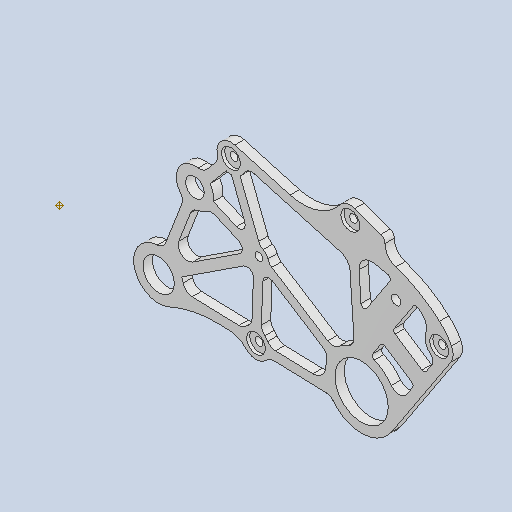
# Autodesk Inventor part: ギア抑え
Saved by Autodesk Inventor 2023 (Build 270158000, 158)
## iProperties
Created: 2022-01-29
Part Number: ギア抑え
Material: Aluminum 2014-T6
Document SubType Name: Modeling
Designer: acps
Density: 2.78927 g/cm^3
Appearance: Satin
Author: acps
Autodesk Inventor part; units mm, degrees
ref_plane "YZ Plane" through (0, 0, 0) normal (1, 0, 0) x (0, 1, 0)
ref_plane "XZ Plane" through (0, 0, 0) normal (0, 1, 0) x (-1, 0, 0)
ref_plane "XY Plane" through (0, 0, 0) normal (0, 0, 1) x (1, 0, 0)
sketch "Sketch4" plane through (0, 0, 0) normal (0, 0, 1) x (1, 0, 0)
  circle A0 centre (58.1571, 43.8132) radius 1.25
  circle A1 centre (46.616, 30) radius 3
  circle A2 centre (35, 0) radius 5.025
  circle A3 centre (67.0906, 21) radius 1.25
  circle A4 centre (67.0906, 21) radius 3
  circle A5 centre (66.1789, -3.483) radius 1.25
  circle A6 centre (58.1571, 43.8132) radius 4.5
  circle A7 centre (66.1789, -3.483) radius 4.5
  circle A8 centre (46.616, 30) radius 6
  circle A9 centre (100, 0) radius 8.525
  circle A10 centre (124.8574, 25) radius 1.25
  circle A11 centre (124.8574, 25) radius 4.5
  circle A12 centre (100, 0) radius 11.525
  circle A13 centre (35, 0) radius 8.025
  line L0 (59.3787, 48.1442) -> (77.1194, 43.1404)
  line L1 (128.6167, 22.5266) -> (109.628, -6.3346)
  line L2 (122.5484, 18.7615) -> (114.5052, 6.5365)
  line L3 (100.7071, 11.5033) -> (100.7003, 11.6011) construction
  line L4 (97.7142, 11.2961) -> (97.7075, 11.3939) construction
  line L5 (68.4738, 18.3379) -> (68.492, 18.3263) construction
  line L6 (70.0876, 20.8669) -> (71.243, 20.1297) construction
  line L7 (67.0906, 21) -> (100, 0) construction
  line L8 (67.0906, 21) -> (124.8574, 25) construction
  line L9 (105.9328, 11.9634) -> (90.1084, 10.8677) construction
  line L10 (100, 0) -> (97.2271, 40.0448) construction
  line L11 (65.705, -7.958) -> (65.6864, -7.956) construction
  line L12 (65.6964, -7.9837) -> (66.1849, -7.983) construction
  line L13 (65.4949, 18.4595) -> (65.4836, 18.1558) construction
  line L14 (67.8357, 0.7009) -> (67.9011, 2.457) construction
  line L15 (67.0906, 21) -> (66.1789, -3.483) construction
  arc A14 (71.4365, 16.4474) -> (68.3621, 14.8358) centre (70.3607, 14.7614) ccw
  line L16 (68.492, 18.3263) -> (68.4928, 18.3479) construction
  line L17 (68.492, 18.3263) -> (71.4365, 16.4474) construction
  line L18 (35, 0) -> (46.616, 30) construction
  line L19 (43.1196, 25.1241) -> (42.4029, 23.2732) construction
  line L20 (39.2454, 6.8101) -> (41.4547, 12.5158) construction
  line L21 (46.616, 30) -> (67.0906, 21) construction
  line L22 (51.3308, 26.289) -> (53.1477, 25.4903) construction
  line L23 (52.538, 29.0354) -> (59.937, 25.783)
  line L24 (61.1008, 40.4096) -> (67.0402, 25.2423)
  line L25 (67.0906, 21) -> (58.1571, 43.8132) construction
  line L26 (58.3073, 39.3157) -> (62.6041, 28.3432)
  arc A15 (59.937, 25.783) -> (62.6041, 28.3432) centre (60.7418, 27.6139) ccw
  line L27 (62.6041, 28.3432) -> (64.7465, 22.8723) construction
  line L28 (59.937, 25.783) -> (65.3157, 23.4187) construction
  line L29 (71.4365, 16.4474) -> (87.5511, 6.1645)
  line L30 (68.3621, 14.8358) -> (68.492, 18.3263) construction
  line L31 (46.616, 30) -> (58.1571, 43.8132) construction
  line L32 (51.492, 33.4964) -> (56.5879, 39.5957)
  line L33 (49.1898, 35.4199) -> (50.4624, 36.943) construction
  arc A16 (58.9156, 37.7626) -> (55.5184, 38.3156) centre (57.0532, 37.0333) ccw
  line L34 (35, 0) -> (67.0906, 21) construction
  line L35 (40.7753, 5.572) -> (45.895, 8.9223) construction
  line L36 (65.738, 18.3222) -> (62.2459, 16.037) construction
  arc A17 (60.8674, 18.7202) -> (60.577, 22.2246) centre (59.7722, 20.3937) ccw
  line L37 (60.577, 22.2246) -> (64.1085, 20.6723) construction
  line L38 (60.8674, 18.7202) -> (64.0952, 20.8325) construction
  arc A18 (65.3396, 14.2891) -> (62.2459, 16.037) centre (63.341, 14.3635) ccw
  line L39 (62.2459, 16.037) -> (42.418, 3.0617)
  line L40 (65.3396, 14.2891) -> (64.9032, 2.5686)
  line L41 (65.4836, 18.1558) -> (65.3396, 14.2891) construction
  circle A19 centre (58.1571, 43.8132) radius 3.025
  circle A20 centre (124.8574, 25) radius 3.025
  circle A21 centre (66.1789, -3.483) radius 3.025
  line L42 (42.994, -0.7047) -> (45.7073, -0.79) construction
  line L43 (70.5412, -2.3784) -> (72.4006, -2.4369) construction
  line L44 (62.6476, 44.1052) -> (65.6368, 43.262) construction
  arc A22 (118.6753, 31.9015) -> (102.5834, 37.8093) centre (98.9344, 3) ccw
  arc A23 (120.5723, 26.3742) -> (118.6753, 31.9015) centre (115.9192, 27.8664) ccw
  arc A24 (103.7268, 37.6704) -> (99.1887, 33.4317) centre (103.1791, 33.708) ccw
  arc A25 (77.1194, 43.1404) -> (93.0418, 48.3811) centre (81.1913, 57.5771) ccw
  circle A26 centre (96.3994, 45.7756) radius 1.25
  circle A27 centre (96.3994, 45.7756) radius 4.25
  arc A28 (122.5484, 18.7615) -> (122.1022, 21.4421) centre (120.8776, 19.8608) ccw
  arc A29 (109.5207, 6.4948) -> (114.5052, 6.5365) centre (111.999, 8.1854) ccw
  line L45 (114.5052, 6.5365) -> (111.3846, 1.7934) construction
  arc A30 (84.3946, -2.8136) -> (88.5086, 0.8792) centre (84.5202, 1.1844) ccw
  line L46 (84.3946, -2.8136) -> (88.86, -2.9539) construction
  arc A31 (107.4852, 44.8614) -> (110.9454, 40.1044) centre (112.4852, 44.8614) ccw
  arc A32 (124.964, 32.0424) -> (110.9454, 40.1044) centre (98.9344, 3) ccw
  arc A33 (128.8264, 27.1206) -> (124.964, 32.0424) centre (112.9503, 18.6382) ccw
  line L47 (97.8537, 49.769) -> (106.1696, 46.7406)
  arc A34 (107.4852, 44.8614) -> (106.1696, 46.7406) centre (105.4852, 44.8614) ccw
  arc A35 (41.4547, 12.5158) -> (45.895, 8.9223) centre (44.2523, 11.4326) ccw
  line L48 (41.4547, 12.5158) -> (45.2005, 22.19)
  line L49 (45.895, 8.9223) -> (60.8674, 18.7202)
  arc A36 (42.8623, 1.6076) -> (45.7073, -0.79) centre (45.8015, 2.2085) ccw
  line L50 (45.7073, -0.79) -> (60.6999, -1.261)
  arc A37 (34.5908, 8.0146) -> (37.2354, 9.9274) centre (34.4378, 11.0107) ccw
  line L51 (37.2354, 9.9274) -> (36.4478, 7.8933) construction
  arc A38 (42.4029, 23.2732) -> (41.9422, 26.2376) centre (39.6053, 24.3565) ccw
  line L52 (42.4029, 23.2732) -> (37.2354, 9.9274)
  arc A39 (47.6454, 35.911) -> (50.4624, 36.943) centre (48.1601, 38.8666) ccw
  line L53 (50.4624, 36.943) -> (53.159, 40.1706)
  arc A40 (65.6368, 43.262) -> (62.1563, 41.7501) centre (64.8224, 40.3747) ccw
  line L54 (65.6368, 43.262) -> (93.3856, 35.4353)
  arc A41 (60.6999, -1.261) -> (62.948, -0.3507) centre (60.7941, 1.7376) ccw
  line L55 (60.6999, -1.261) -> (62.2387, -1.3093) construction
  arc A42 (69.9684, -1.0562) -> (72.4006, -2.4369) centre (72.4948, 0.5617) ccw
  line L56 (72.4006, -2.4369) -> (84.3946, -2.8136)
  arc A43 (63.6147, 0.2149) -> (64.9032, 2.5686) centre (61.9053, 2.6803) ccw
  arc A44 (67.9011, 2.457) -> (69.011, 0.014) centre (70.899, 2.3454) ccw
  line L57 (64.9032, 2.5686) -> (64.8378, 0.8125) construction
  line L58 (67.9011, 2.457) -> (68.3621, 14.8358)
  arc A45 (67.0402, 25.2423) -> (68.4621, 23.6681) centre (69.8336, 26.3362) ccw
  arc A46 (69.9736, 21.8293) -> (71.243, 20.1297) centre (72.8567, 22.6586) ccw
  line L59 (67.0402, 25.2423) -> (67.5399, 23.9662) construction
  line L60 (71.243, 20.1297) -> (89.1649, 8.6934)
  arc A47 (53.159, 40.1706) -> (53.7769, 42.7817) centre (50.8568, 42.0941) ccw
  line L61 (53.159, 40.1706) -> (54.2857, 41.5192) construction
  arc A48 (47.5374, 24.0712) -> (45.2005, 22.19) centre (47.9981, 21.1068) ccw
  arc A49 (53.1477, 25.4903) -> (50.1657, 25.1626) centre (51.9405, 22.744) ccw
  line L62 (45.2005, 22.19) -> (45.9172, 24.0408) construction
  line L63 (53.1477, 25.4903) -> (60.577, 22.2246)
  arc A50 (96.2902, 31.8619) -> (93.3856, 35.4353) centre (92.2997, 31.5855) ccw
  arc A51 (88.8418, 2.8846) -> (87.5511, 6.1645) centre (85.9373, 3.6355) ccw
  arc A52 (89.1649, 8.6934) -> (92.6832, 8.9045) centre (90.7787, 11.2224) ccw
  arc A53 (95.681, 10.6851) -> (97.5496, 13.6737) centre (94.5568, 13.4665) ccw
  arc A54 (100.5424, 13.881) -> (102.8051, 11.1784) centre (103.5353, 14.0882) ccw
  line L64 (87.5511, 6.1645) -> (89.5603, 4.8824) construction
  line L65 (89.1649, 8.6934) -> (91.174, 7.4113) construction
  line L66 (97.7075, 11.3939) -> (97.5496, 13.6737) construction
  line L67 (97.5496, 13.6737) -> (96.2902, 31.8619)
  line L68 (100.7003, 11.6011) -> (100.5424, 13.881) construction
  line L69 (100.5424, 13.881) -> (99.1887, 33.4317)
  circle A55 centre (111.0805, 30.9772) radius 1.5
  arc A56 (109.045, 35.1608) -> (108.4824, 36.6725) centre (108.2096, 35.7104) ccw
  arc A57 (117.9732, 32.3688) -> (116.5938, 32.0793) centre (117.4292, 31.5297) ccw
  line L70 (109.045, 35.1608) -> (101.6472, 23.9169)
  line L71 (116.5938, 32.0793) -> (103.5648, 12.2763)
  arc A58 (103.5648, 12.2763) -> (104.0488, 10.7904) centre (104.4002, 11.7266) ccw
  arc A59 (99.8142, 24.3974) -> (101.6472, 23.9169) centre (100.8118, 24.4665) ccw
  arc A60 (107.4624, 16.381) -> (106.0773, 16.0952) centre (106.9127, 15.5456) ccw
  line L72 (107.4624, 16.381) -> (116.0624, 10.7227)
  arc A61 (116.3482, 9.3377) -> (116.0624, 10.7227) centre (115.5128, 9.8873) ccw
  line L73 (111.877, 28.1536) -> (124.7416, 19.6896) construction
  line L74 (107.3053, 20.0754) -> (119.422, 12.1035) construction
  line L75 (110.7602, 21.3934) -> (119.3603, 15.7351)
  arc A62 (110.4744, 22.7784) -> (110.7602, 21.3934) centre (111.3098, 22.2288) ccw
  arc A63 (119.3603, 15.7351) -> (120.7453, 16.0209) centre (119.9099, 16.5705) ccw
  line L76 (102.8536, 11.9183) -> (111.9722, 5.9189) construction
  circle A64 centre (96.3994, 45.7756) radius 3.025
  arc A65 (56.821, -6.4645) -> (37.4687, -8.6808) centre (53.881, -66.3925) ccw construction
  arc A66 (56.821, -6.4645) -> (59.8142, -6.4542) centre (58.2196, 22.0427) ccw construction
  arc A67 (71.3782, -23.4684) -> (59.8142, -6.4542) centre (60.4847, -18.4355) ccw construction
  arc A68 (54.4173, -4.0651) -> (38.3334, -7.2999) centre (53.2869, -40.0473) ccw
  line L77 (54.4173, -4.0651) -> (57.8446, -4.1727)
  arc A69 (62.8316, -6.4907) -> (57.8446, -4.1727) centre (57.6249, -11.1693) ccw
  arc A70 (71.9175, -5.4232) -> (69.5655, -6.4462) centre (71.8233, -8.4217) ccw
  line L78 (71.9175, -5.4232) -> (88.6522, -5.9489)
  arc A71 (90.9212, -7.0994) -> (88.6522, -5.9489) centre (88.558, -8.9474) ccw
  point P0 (0, 0)
  point P1 (62.6167, 23.75)
  point P2 (63.8469, 21.7439)
  point P3 (63.7276, 4.995)
  point P4 (48.9428, 29.7841)
  point P5 (49.819, 30.1472)
  point P6 (62.9071, 26.3997)
  point P7 (50.9368, 32.3834)
  point P8 (50.8115, 33.0283)
  point P9 (57.8297, 40.9724)
  point P10 (62.9138, 26.4056)
  point P11 (67.612, 23.8643)
  point P12 (65.579, 26.356)
  point P13 (60.2796, 41.5397)
  point P14 (109.8309, 27.4562)
  point P15 (109.8687, 27.322)
  point P16 (93.5994, 9.6725)
  point P17 (91.8321, 9.416)
  point P18 (89.3299, 7.9976)
  point P19 (66.2271, 4.9132)
  point P20 (66.3467, 21.7081)
  point P21 (48.9379, 34.6835)
  point P22 (46.5685, 30.5773)
  point P23 (64.7751, 2.2487)
  point P24 (65.1323, 2.2448)
  point P25 (91.0705, 5.7078)
  point P26 (95.4376, 7.978)
  point P27 (111.7069, 25.6275)
  point P28 (110.5144, 29.861)
  point P29 (60.7307, 44.0105)
  point P30 (55.9361, 42.605)
  point P31 (92.4107, 6.1598)
  point P32 (92.438, 8.4126)
  point P33 (93.6914, 8.3068)
  point P34 (64.5533, 22.7819)
  point P35 (64.4718, 22.8265)
  point P36 (65.6711, 25.0181)
  point P37 (47.5045, 33.0609)
  point P38 (49.0002, 33.3514)
  point P39 (49.5268, 31.5741)
  point P40 (62.6167, 23.75)
  point P41 (63.8469, 21.7439)
  point P42 (63.7276, 4.995)
  point P43 (48.9428, 29.7841)
  point P44 (49.819, 30.1472)
  point P45 (62.9071, 26.3997)
  point P46 (50.9368, 32.3834)
  point P47 (50.8115, 33.0283)
  point P48 (57.8297, 40.9724)
  point P49 (62.9138, 26.4056)
  point P50 (67.612, 23.8643)
  point P51 (65.579, 26.356)
  point P52 (60.2796, 41.5397)
  point P53 (109.8309, 27.4562)
  point P54 (109.8687, 27.322)
  point P55 (93.5994, 9.6725)
  point P56 (91.8321, 9.416)
  point P57 (89.3299, 7.9976)
  point P58 (66.2271, 4.9132)
  point P59 (66.3467, 21.7081)
  point P60 (48.9379, 34.6835)
  point P61 (46.5685, 30.5773)
  point P62 (64.7751, 2.2487)
  point P63 (65.1323, 2.2448)
  point P64 (91.0705, 5.7078)
  point P65 (95.4376, 7.978)
  point P66 (111.7069, 25.6275)
  point P67 (110.5144, 29.861)
  point P68 (60.7307, 44.0105)
  point P69 (55.9361, 42.605)
  point P70 (92.4107, 6.1598)
  point P71 (92.438, 8.4126)
  point P72 (93.6914, 8.3068)
  point P73 (64.5533, 22.7819)
  point P74 (64.4718, 22.8265)
  point P75 (65.6711, 25.0181)
  point P76 (47.5045, 33.0609)
  point P77 (49.0002, 33.3514)
  point P78 (49.5268, 31.5741)
  point P79 (62.6167, 23.75)
  point P80 (63.8469, 21.7439)
  point P81 (63.7276, 4.995)
  point P82 (48.9428, 29.7841)
  point P83 (49.819, 30.1472)
  point P84 (62.9071, 26.3997)
  point P85 (50.9368, 32.3834)
  point P86 (50.8115, 33.0283)
  point P87 (57.8297, 40.9724)
  point P88 (62.9138, 26.4056)
  point P89 (67.612, 23.8643)
  point P90 (65.579, 26.356)
  point P91 (60.2796, 41.5397)
  point P92 (109.8309, 27.4562)
  point P93 (109.8687, 27.322)
  point P94 (93.5994, 9.6725)
  point P95 (91.8321, 9.416)
  point P96 (89.3299, 7.9976)
  point P97 (66.2271, 4.9132)
  point P98 (66.3467, 21.7081)
  point P99 (48.9379, 34.6835)
  point P100 (46.5685, 30.5773)
  point P101 (64.7751, 2.2487)
  point P102 (65.1323, 2.2448)
  point P103 (91.0705, 5.7078)
  point P104 (95.4376, 7.978)
  point P105 (111.7069, 25.6275)
  point P106 (110.5144, 29.861)
  point P107 (60.7307, 44.0105)
  point P108 (55.9361, 42.605)
  point P109 (92.4107, 6.1598)
  point P110 (92.438, 8.4126)
  point P111 (93.6914, 8.3068)
  point P112 (64.5533, 22.7819)
  point P113 (64.4718, 22.8265)
  point P114 (65.6711, 25.0181)
  point P115 (47.5045, 33.0609)
  point P116 (49.0002, 33.3514)
  point P117 (49.5268, 31.5741)
  point P118 (62.6167, 23.75)
  point P119 (63.8469, 21.7439)
  point P120 (63.7276, 4.995)
  point P121 (48.9428, 29.7841)
  point P122 (49.819, 30.1472)
  point P123 (62.9071, 26.3997)
  point P124 (50.9368, 32.3834)
  point P125 (50.8115, 33.0283)
  point P126 (57.8297, 40.9724)
  point P127 (62.9138, 26.4056)
  point P128 (67.612, 23.8643)
  point P129 (65.579, 26.356)
  point P130 (60.2796, 41.5397)
  point P131 (109.8309, 27.4562)
  point P132 (109.8687, 27.322)
  point P133 (93.5994, 9.6725)
  point P134 (91.8321, 9.416)
  point P135 (89.3299, 7.9976)
  point P136 (66.2271, 4.9132)
  point P137 (66.3467, 21.7081)
  point P138 (48.9379, 34.6835)
  point P139 (46.5685, 30.5773)
  point P140 (64.7751, 2.2487)
  point P141 (65.1323, 2.2448)
  point P142 (91.0705, 5.7078)
  point P143 (95.4376, 7.978)
  point P144 (111.7069, 25.6275)
  point P145 (110.5144, 29.861)
  point P146 (60.7307, 44.0105)
  point P147 (55.9361, 42.605)
  point P148 (92.4107, 6.1598)
  point P149 (92.438, 8.4126)
  point P150 (93.6914, 8.3068)
  point P151 (64.5533, 22.7819)
  point P152 (64.4718, 22.8265)
  point P153 (65.6711, 25.0181)
  point P154 (47.5045, 33.0609)
  point P155 (49.0002, 33.3514)
  point P156 (49.5268, 31.5741)
  point P157 (62.6167, 23.75)
  point P158 (63.8469, 21.7439)
  point P159 (63.7276, 4.995)
  point P160 (48.9428, 29.7841)
  point P161 (49.819, 30.1472)
  point P162 (62.9071, 26.3997)
  point P163 (50.9368, 32.3834)
  point P164 (50.8115, 33.0283)
  point P165 (57.8297, 40.9724)
  point P166 (62.9138, 26.4056)
  point P167 (67.612, 23.8643)
  point P168 (65.579, 26.356)
  point P169 (60.2796, 41.5397)
  point P170 (109.8309, 27.4562)
  point P171 (109.8687, 27.322)
  point P172 (93.5994, 9.6725)
  point P173 (91.8321, 9.416)
  point P174 (89.3299, 7.9976)
  point P175 (66.2271, 4.9132)
  point P176 (66.3467, 21.7081)
  point P177 (48.9379, 34.6835)
  point P178 (46.5685, 30.5773)
  point P179 (64.7751, 2.2487)
  point P180 (65.1323, 2.2448)
  point P181 (91.0705, 5.7078)
  point P182 (95.4376, 7.978)
  point P183 (111.7069, 25.6275)
  point P184 (110.5144, 29.861)
  point P185 (60.7307, 44.0105)
  point P186 (55.9361, 42.605)
  point P187 (92.4107, 6.1598)
  point P188 (92.438, 8.4126)
  point P189 (93.6914, 8.3068)
  point P190 (64.5533, 22.7819)
  point P191 (64.4718, 22.8265)
  point P192 (65.6711, 25.0181)
  point P193 (47.5045, 33.0609)
  point P194 (49.0002, 33.3514)
  point P195 (49.5268, 31.5741)
  point P196 (67.0906, 21)
  point P197 (110.4744, 22.7784)
  point P198 (120.7453, 16.0209)
  dimension "d526" = 6
  dimension "d528" = 9
  dimension "d529" = 9
  dimension "d522" = 2.5
  dimension "d523" = 6
  dimension "d524" = 10.05
  dimension "d525" = 2.5
  dimension "d527" = 2.5
  dimension "d530" = 3
  dimension "d531" = 17.05
  dimension "d532" = 2.5
  dimension "d533" = 9
  dimension "d534" = 3
  dimension "d535" = 3
  dimension "d536" = 3
  dimension "d537" = 3
  dimension "d538" = 3
  dimension "d539" = 1.5
  dimension "d540" = 1.5
  dimension "d541" = 3
  dimension "d542" = 1.5
  dimension "d543" = 2
  dimension "d544" = 3
  dimension "d545" = 1.5
  dimension "d546" = 3
  dimension "d547" = 1.5
  dimension "d548" = 3
  dimension "d549" = 1.5
  dimension "d550" = 2
  dimension "d551" = 3
  dimension "d552" = 1.5
  dimension "d553" = 2
  dimension "d554" = 3
  dimension "d555" = 1.5
  dimension "d556" = 2
  dimension "d557" = 2
  dimension "d558" = 6.05
  dimension "d559" = 6.05
  dimension "d560" = 6.05
  dimension "d561" = 3
  dimension "d562" = 4
  dimension "d563" = 3
  dimension "d564" = 15
  dimension "d565" = 2
  dimension "d566" = 3
  dimension "d567" = 4
  dimension "d568" = 18
  dimension "d569" = 2
  dimension "d570" = 3
  dimension "d571" = 3
  dimension "d572" = 3
  dimension "d573" = 3
  dimension "d574" = 3
  dimension "d575" = 3
  dimension "d576" = 3
  dimension "d577" = 3
  dimension "d578" = 3
  dimension "d579" = 3
  dimension "d580" = 3
  dimension "d581" = 3
  dimension "d582" = 3
  dimension "d583" = 3
  dimension "d584" = 3
  dimension "d585" = 4
  dimension "d586" = 3
  dimension "d587" = 3
  dimension "d588" = 3
  constraints: 158 end point, 117 tangent, 111 point on circle, 97 parallel, 66 centre point, 15 coincident, 11 point on line, 8 perpendicular, 6 symmetric about line, 1 concentric, 128 other
  measures "d522" diameter of A0
  measures "d523" diameter of A1
  measures "d524" diameter of A2
  measures "d525" diameter of A3
  measures "d527" diameter of A5
  measures "d530" radius of A1
  measures "d531" diameter of A9
  measures "d532" diameter of A10
  measures "d533" diameter of A11
  measures "d536" distance between parallel lines of L1 L2
  measures "d537" distance between parallel lines of L3 L4
  measures "d538" distance between parallel lines of L5 L6
  measures "d539" distance between parallel lines of L6 L7
  measures "d540" distance between parallel lines of L10 L4
  measures "d541" distance between parallel lines of L13 L14
  measures "d542" distance between parallel lines of L13 L15
  measures "d543" radius of A14
  measures "d544" distance between parallel lines of L19 L20
  measures "d545" distance between parallel lines of L18 L20
  measures "d546" distance between parallel lines of L22 L23
  measures "d547" distance between parallel lines of L22 L21
  measures "d548" distance between parallel lines of L26 L24
  measures "d549" distance between parallel lines of L24 L25
  measures "d550" radius of A15
  measures "d551" distance between parallel lines of L33 L32
  measures "d552" distance between parallel lines of L31 L32
  measures "d553" radius of A16
  measures "d554" distance between parallel lines of L35 L36
  measures "d555" distance between parallel lines of L36 L34
  measures "d556" radius of A17
  measures "d557" radius of A18
  measures "d558" diameter of A19
  measures "d559" diameter of A20
  measures "d560" diameter of A21
  measures "d561" distance between parallel lines of L44 L0
  measures "d562" radius of A24
  measures "d563" radial gap between concentric circles of A26 A27
  measures "d564" radius of A25
  measures "d565" radius of A28
  measures "d566" radius of A29
  measures "d567" radius of A30
  measures "d568" radius of A33
  measures "d569" radius of A34
  measures "d570" radius of A35
  measures "d571" radius of A36
  measures "d572" radius of A37
  measures "d573" radius of A38
  measures "d574" radius of A39
  measures "d575" radius of A40
  measures "d576" radius of A41
  measures "d577" radius of A42
  measures "d578" radius of A43
  measures "d579" radius of A44
  measures "d580" radius of A45
  measures "d581" radius of A46
  measures "d582" radius of A47
  measures "d583" radius of A48
  measures "d584" radius of A49
  measures "d585" radius of A50
  measures "d586" radius of A51
  measures "d587" radius of A52
  measures "d588" radius of A53
extrude "Extrusion3" add sketch "Sketch4" along normal blind 3 contours A4 | A4 A46 L60 A52 A12 A51 L29 A14 L58 A44 A7 A43 L40 A18 L39 A13 A37 L52 A38 A8 A48 L48 A35 L49 A17 L63 A49 L23 A15 L26 A6 L24 A45 | A6 | A12 | A6 L0 A25 A27 L47 A34 A31 A32 A33 A11 A23 A22 A24 L69 A54 A12 A53 L67 A50 L54 A40 | L32 A8 A39 L53 A47 A6 | A54 L69 A59 L70 A56 A22 A57 L71 A58 A12 | A12 A71 L78 A70 A7 A42 L56 A30 | A8 | A29 L2 A28 A11 L1 A12 | A27 | L71 A62 L75 A63 L2 A61 L72 A60 | A11 | A7 | A69 L77 A68 A13 A36 L50 A41 A7 | A13
extrude "押し出し6" add sketch "Sketch4" along normal blind 2 contours A19 | A20 | A21 | A64
body "Solid2"
